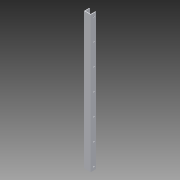
# Autodesk Inventor part: 26in C-Channel Left
Saved by Autodesk Inventor 2013 (Build 170138000, 138)
## iProperties
Created: 2013-01-08
Part Number: 26in C-Channel Left
Material: Aluminum 6061
Document SubType Name: Modeling
Designer: Naphat
Density: 1 g/cm^3
Author: Naphat
Autodesk Inventor part; units mm, degrees
ref_plane "YZ Plane" through (0, 0, 0) normal (1, 0, 0) x (0, 1, 0)
ref_plane "XZ Plane" through (0, 0, 0) normal (0, 1, 0) x (-1, 0, 0)
ref_plane "XY Plane" through (0, 0, 0) normal (0, 0, 1) x (1, 0, 0)
sketch "Sketch1" plane through (0, 0, 0) normal (0, 0, 1) x (1, 0, 0)
  line L0 (-16, 12.5) -> (-13, 12.5)
  line L1 (-13, 12.5) -> (-13, -9.5)
  line L2 (-13, -9.5) -> (13, -9.5)
  line L3 (13, -9.5) -> (13, 12.5)
  line L4 (13, 12.5) -> (16, 12.5)
  line L5 (16, 12.5) -> (16, -12.5)
  line L6 (16, -12.5) -> (-16, -12.5)
  line L7 (-16, -12.5) -> (-16, 12.5)
  point P0 (0, 0)
  dimension "d0" = 3
  dimension "d2" = 3
  dimension "d3" = 25
  dimension "d4" = 32
  dimension "d5" = 16
  dimension "d7" = 12.5
  dimension "d8" = 3
  dimension "d95" = 25
  constraints: 16 end point, 5 parallel, 1 collinear, 1 horizontal, 1 perpendicular
  measures "d0" distance of L0.start L0.end
  measures "d2" distance of L3.end L4.end
  measures "d3" distance of L6.end L0.start
  measures "d4" distance of L5.end L6.end
  measures "d5" distance from line of point (0, 0) L7
  measures "d7" distance from line of L6 point (0, 0)
  measures "d8" distance between parallel lines of L6 L2
  measures "d95" distance between parallel lines of L6 L4
extrude "Extrusion1" add sketch "Sketch1" against normal blind 660.4
sketch "Sketch5" plane through (16, -12.5, 0) normal (1, 0, 0) x (0, 0, -1)
  circle A0 centre (16, 15.5) radius 3.175
  circle A1 centre (120.7333, 15.5) radius 3.175
  circle A2 centre (225.4667, 15.5) radius 3.175
  circle A3 centre (330.2, 15.5) radius 3.175
  circle A4 centre (434.9333, 15.5) radius 3.175
  circle A5 centre (539.6667, 15.5) radius 3.175
  circle A6 centre (644.4, 15.5) radius 3.175
  line L0 (0, 25) -> (0, 0) projected
  line L1 (660.4, 25) -> (660.4, 0) projected
  line L2 (0, 3) -> (660.4, 3) projected
  point P0 (0, 12.5)
  dimension "d56" = 6.35
  dimension "d58" = 6.35
  dimension "d59" = 6.35
  dimension "d61" = 6.35
  dimension "d63" = 6.35
  dimension "d64" = 6.35
  dimension "d65" = 6.35
  dimension "d68" = 16
  dimension "d78" = 660.4
  dimension "d79" = 16
  dimension "d80" = 628.4
  dimension "d81" = 104.7333
  dimension "d82" = 104.7333
  dimension "d83" = 104.7333
  dimension "d84" = 104.7333
  dimension "d85" = 104.7333
  dimension "d86" = 104.7333
  dimension "d94" = 12.5
  constraints: 7 centre point, 6 horizontal alignment
  measures "d56" diameter of A0
  measures "d58" diameter of A1
  measures "d59" diameter of A2
  measures "d61" diameter of A3
  measures "d63" diameter of A4
  measures "d64" diameter of A5
  measures "d65" diameter of A6
  measures "d68" distance from line of L1 A6.centre
  measures "d78" distance of L0.end L1.end
  measures "d79" distance from line of A0.centre L0
  measures "d80" distance of A6.centre A0.centre
  measures "d81" distance of A6.centre A5.centre
  measures "d82" distance of A5.centre A4.centre
  measures "d83" distance of A4.centre A3.centre
  measures "d84" distance of A3.centre A2.centre
  measures "d85" distance of A2.centre A1.centre
  measures "d86" distance of A1.centre A0.centre
  measures "d94" distance from line of L2 A6.centre
hole "Hole1" at (16, 3, -644.4) at (16, 3, -539.6667) at (16, 3, -434.9333) at (16, 3, -330.2) at (16, 3, -225.4667) at (16, 3, -120.7333) at (16, 3, -16) direction (-1, 0, 0) diameter 6.35 depth 3 tip angle 118
sketch "Sketch6" plane through (-16, -12.5, 0) normal (-1, 0, 0) x (0, 0, 1)
  circle A0 centre (-16, 15.5) radius 3.175 projected
  circle A1 centre (-644.4, 15.5) radius 3.175 projected
  circle A2 centre (-644.4, 15.5) radius 3.175
  circle A3 centre (-16, 15.5) radius 3.175
  point P0 (0, 12.5)
  constraints: 2 centre point, 2 coincident, 2 concentric
hole "Hole2" at (-16, 3, -644.4) at (-16, 3, -16) direction (1, 0, 0) diameter 6.35 depth 3 tip angle 118
equation "\"d2\" = d0"
equation "\"d5\" = 0.5 * d4"
equation "\"d7\" = 0.5 * d3"
equation "\"d8\" = d0"
equation "\"d95\" = d3"
equation "\"d58\" = d56"
equation "\"d59\" = d58"
equation "\"d61\" = d60"
equation "\"d63\" = d62"
equation "\"d64\" = d63"
equation "\"d65\" = d64"
equation "\"d81\" = 0.166667 * d80"
equation "\"d82\" = d81"
equation "\"d83\" = d82"
equation "\"d84\" = d83"
equation "\"d85\" = d84"
equation "\"d60\" = d59"
equation "\"d62\" = d61"
body "Solid1"
